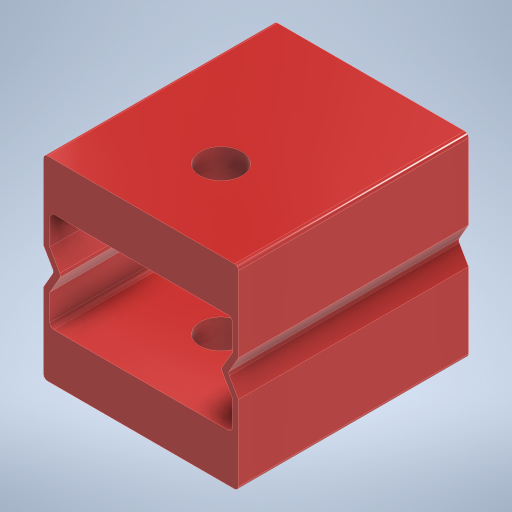
# Autodesk Inventor part: X_belt2
Saved by Autodesk Inventor 2023 (Build 270158000, 158)
## iProperties
Created: 2023-03-07
Part Number: X_belt2
Material: Типовые
Document SubType Name: Modeling
Designer: Josh
Density: 1 g/cm^3
Appearance: Оранжево-красный
Author: Josh
Autodesk Inventor part; units mm, degrees
ref_plane "YZ Plane" through (0, 0, 0) normal (1, 0, 0) x (0, 1, 0)
ref_plane "XZ Plane" through (0, 0, 0) normal (0, 1, 0) x (-1, 0, 0)
ref_plane "XY Plane" through (0, 0, 0) normal (0, 0, 1) x (1, 0, 0)
sketch "Эскиз1" plane through (0, 0, 0) normal (0, 0, 1) x (1, 0, 0)
  line L0 (10, -10) -> (-10, -10) construction
  line L1 (-10, -10) -> (-10, -1.7321) construction
  line L2 (-10, 10) -> (10, 10) construction
  line L3 (10, 10) -> (10, 1.7321) construction
  line L4 (10, -10) -> (-10, 10) construction
  line L5 (-10, -10) -> (10, 10) construction
  line L6 (-10, 1.7321) -> (-9, 0) construction
  line L7 (-9, 0) -> (-10, -1.7321) construction
  line L8 (0, 10) -> (0, -10)
  line L9 (10, 1.7321) -> (9, 0) construction
  line L10 (9, 0) -> (10, -1.7321) construction
  line L11 (-10, 1.7321) -> (-10, 10) construction
  line L12 (-10, -1.7321) -> (-10, 1.7321) construction
  line L13 (10, 1.7321) -> (10, -1.7321) construction
  line L14 (10, -1.7321) -> (10, -10) construction
  line L15 (9.75, 9.75) -> (-9.75, 9.75)
  line L16 (-9.75, 9.75) -> (-9.75, 1.799)
  line L17 (-9.75, 1.799) -> (-8.7113, 0)
  line L18 (-8.7113, 0) -> (-9.75, -1.799)
  line L19 (-9.75, -1.799) -> (-9.75, -9.75)
  line L20 (-9.75, -9.75) -> (9.75, -9.75)
  line L21 (9.75, -9.75) -> (9.75, -1.799)
  line L22 (9.75, -1.799) -> (8.7113, 0)
  line L23 (8.7113, 0) -> (9.75, 1.799)
  line L24 (9.75, 1.799) -> (9.75, 9.75)
  line L25 (-9.134, 1.9641) -> (-9.134, 9.134)
  line L26 (-9.134, 9.134) -> (9.134, 9.134)
  line L27 (9.134, 9.134) -> (9.134, 1.9641)
  line L28 (9.134, 1.9641) -> (8, 0)
  line L29 (8, 0) -> (9.134, -1.9641)
  line L30 (9.134, -1.9641) -> (9.134, -9.134)
  line L31 (9.134, -9.134) -> (-9.134, -9.134)
  line L32 (-9.134, -9.134) -> (-9.134, -1.9641)
  line L33 (-9.134, -1.9641) -> (-8, 0)
  line L34 (-8, 0) -> (-9.134, 1.9641)
  line L35 (9.134, -5) -> (-9.134, -5)
  line L36 (-9.134, -5) -> (-9.134, -1.9641)
  line L37 (-9.134, 5) -> (9.134, 5)
  line L38 (9.134, 5) -> (9.134, 1.9641)
  line L39 (9.134, -5) -> (-9.134, 5) construction
  line L40 (-9.134, -5) -> (9.134, 5) construction
  line L41 (-9.134, 1.9641) -> (-9.134, 5)
  line L42 (-9.134, -1.9641) -> (-9.134, 1.9641) construction
  line L43 (9.134, 1.9641) -> (9.134, -1.9641) construction
  line L44 (9.134, -1.9641) -> (9.134, -5)
  point P0 (0, 0)
  dimension "d0" = 20
  dimension "d1" = 20
  dimension "d2" = 9
  dimension "d3" = 150
  dimension "d4" = 0.25
  dimension "d5" = 16
  dimension "d6" = 10
  constraints: 90 end point, 30 parallel, 10 perpendicular, 6 midpoint, 3 symmetric about line, 2 horizontal, 1 equal length, 1 horizontal alignment, 1 point on line, 18 other
  measures "d0" distance of L2.start L2.end
  measures "d1" distance of L0.end L2.start
  measures "d2" distance of point (0, 0) L6.end
  measures "d3" angle of L1 L7
  measures "d4" distance between parallel lines of L2 L15
  measures "d5" distance of L28.end L33.end
  measures "d6" distance of L35.end L37.start
extrude "Выдавливание1" add sketch "Эскиз1" along normal blind 20 contours L15 L24 L23 L22 L21 L20 L8 L31 L30 L29 L28 L27 L26 | L8 L26 L25 L34 L33 L32 L31 L20 L19 L18 L17 L16 L15 | L26 L27 L37 L8 | L8 L37 L25 L26 | L35 L30 L31 L8 | L8 L31 L32 L35
sketch "Эскиз2" plane through (-9.75, 9.75, 0) normal (0, 1, 0) x (1, 0, 0)
  line L0 (9.75, 0) -> (9.75, -20)
  line L1 (0.616, -20) -> (18.884, -20) projected
  circle A0 centre (9.75, -12) radius 8
  circle A1 centre (9.75, -12) radius 2.1
  dimension "d9" = 16
  dimension "d10" = 8
  dimension "d11" = 4.2
  constraints: 2 centre point, 2 end point, 1 coincident, 1 midpoint, 1 point on line
  measures "d9" diameter of A0
  measures "d10" distance from line of L1 A0.centre
  measures "d11" diameter of A1
extrude "Выдавливание2" cut sketch "Эскиз2" against normal through all contours A1 L0 | L0 A1
sketch "Эскиз3" plane through (0, 0, 0) normal (0, 0, -1) x (-1, 0, 0)
  line L0 (9.75, -1.799) -> (9.75, -9.75) projected
  line L1 (-9.75, 9.75) -> (9.75, 9.75)
  line L2 (9.75, 9.75) -> (9.75, -9.75)
  line L3 (9.75, -9.75) -> (-9.75, -9.75)
  line L4 (-9.75, -9.75) -> (-9.75, 9.75)
  line L5 (-8.7113, 0) -> (-9.75, 1.799) projected
  line L6 (-9.75, -1.799) -> (-8.7113, 0) projected
  line L7 (9.75, 1.799) -> (8.7113, 0) projected
  line L8 (8.7113, 0) -> (9.75, -1.799) projected
  point P0 (0, 0)
  constraints: 8 end point, 2 parallel, 1 horizontal, 1 perpendicular
extrude "Выдавливание3" add sketch "Эскиз3" along normal blind 3 contours L0 L3 L4 L6 L5 L1 L2 L7 L8
sketch "Эскиз4" plane through (0, 0, 0) normal (0, 0, 1) x (1, 0, 0)
  circle A0 centre (0, 0) radius 2.1
  dimension "d16" = 4.2
  constraints: 1 centre point, 1 coincident
  measures "d16" diameter of A0
extrude "Выдавливание4" cut sketch "Эскиз4" against normal through all
fillet "Сопряжение1" radius 0.4 4 edges at (9.75, -9.75, 8.5) (9.75, 9.75, 8.5) (-9.75, -9.75, 8.5) (-9.75, 9.75, 8.5)
fillet "Сопряжение2" radius 0.4 4 edges at (-9.134, -5, 10) (-9.134, 5, 10) (9.134, 5, 10) (9.134, -5, 10)
fillet "Сопряжение3" radius 0.4 2 edges at (8, 0, 10) (-8, 0, 10)
fillet "Сопряжение4" radius 0.4 2 edges at (-8.7113, 0, 8.5) (8.7113, 0, 8.5)
